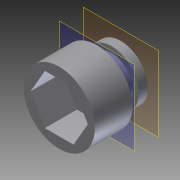
# Autodesk Inventor part: BlankSmallGearOutput
Saved by Autodesk Inventor 2012 (Build 160160000, 160)
## iProperties
Created: 2011-10-26
Part Number: BlankSmallGearOutput
Material: Default
Document SubType Name: Modeling
Designer: akutta
Density: 1 g/cm^3
Author: akutta
Autodesk Inventor part; units mm, degrees
ref_plane "YZ Plane" through (0, 0, 0) normal (1, 0, 0) x (0, 1, 0)
ref_plane "XZ Plane" through (0, 0, 0) normal (0, 1, 0) x (-1, 0, 0)
ref_plane "XY Plane" through (0, 0, 0) normal (0, 0, 1) x (1, 0, 0)
ref_plane "Work Plane3" through (0, 0, 4) normal (0, 0, 1) x (1, 0, 0)
ref_plane "Work Plane4" through (0, 0, 11) normal (0, 0, -1) x (-1, 0, 0)
sketch "Sketch7" plane through (0, 0, 4) normal (0, 0, 1) x (1, 0, 0)
  circle A0 centre (0, 0) radius 3.5
  circle A1 centre (0, 0) radius 7.955
  dimension "d17" = 7
  dimension "d18" = 15.91
  constraints: 2 centre point, 2 coincident
  measures "d17" diameter of A0
  measures "d18" diameter of A1
extrude "Extrusion5" add sketch "Sketch7" along normal blind 2.7 contours A0 | A1
sketch "Sketch8" plane through (0, 0, 6.7) normal (0, 0, 1) x (1, 0, 0)
  circle A0 centre (0, 0) radius 6.25
  dimension "d21" = 12.5
  constraints: 1 centre point, 1 coincident
  measures "d21" diameter of A0
extrude "Extrusion6" add sketch "Sketch8" along normal up to surface (4.3 mm away)
sketch "Sketch9" plane through (0, 0, 11) normal (0, 0, 1) x (1, 0, 0)
  circle A0 centre (0, 0) radius 10.3925
  dimension "d24" = 20.785
  constraints: 1 centre point, 1 coincident
  measures "d24" diameter of A0
extrude "Extrusion7" add sketch "Sketch9" along normal blind 11
sketch "Sketch10" plane through (0, 0, 22) normal (0, 0, 1) x (1, 0, 0)
  circle A0 centre (0, 0) radius 10.3925 projected
  line L0 (-4.1858, 7.25) -> (4.1858, 7.25)
  line L1 (4.1858, 7.25) -> (8.3716, 0)
  line L2 (8.3716, 0) -> (4.1858, -7.25)
  line L3 (4.1858, -7.25) -> (-4.1858, -7.25)
  line L4 (-4.1858, -7.25) -> (-8.3716, 0)
  line L5 (-8.3716, 0) -> (-4.1858, 7.25)
  line L6 (0, 0) -> (4.1858, 7.25) construction
  line L7 (0, 0) -> (8.3716, 0) construction
  line L8 (0, 0) -> (-4.1858, -7.25) construction
  line L9 (-14.5495, 0) -> (14.5495, 0) projected
  dimension "d27" = 14.5
  constraints: 18 end point, 6 equal length, 2 parallel, 2 point on line, 1 horizontal
  measures "d27" distance between parallel lines of L3 L0
extrude "Extrusion8" cut sketch "Sketch10" against normal blind 9.4 contours L9 L5 L0 L1 | L2 L3 L4 L9
body "Solid1"
